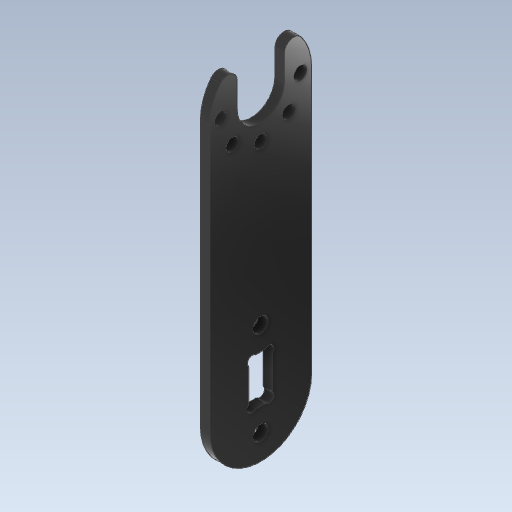
# Autodesk Inventor part: ForeArm_inside_frame
Saved by Autodesk Inventor 2020 (Build 240168000, 168)
## iProperties
Part Number: ForeArm_inside_frame
Material: GFRP
Document SubType Name: Modeling
Designer: Masato Kubotera
Density: 1.75 g/cm^3
Appearance: 低 光沢 - 黒
Description: GFRP T2
Mass: 4.75794 g
Surface Area: 33.053 cm^2
Volume: 2.71883 cm^3
Author: Masato Kubotera
Autodesk Inventor part; units mm, degrees
ref_plane "YZ Plane" through (0, 0, 0) normal (1, 0, 0) x (0, 1, 0)
ref_plane "XZ Plane" through (0, 0, 0) normal (0, 1, 0) x (-1, 0, 0)
ref_plane "XY Plane" through (0, 0, 0) normal (0, 0, 1) x (1, 0, 0)
derived "ForeArm_outside_frame.ipt"
sketch "スケッチ1" plane through (0, 0, 0) normal (0, 1, 0) x (-1, 0, 0)
  circle A0 centre (0, 0) radius 5.05
  line L0 (-8.5, 0) -> (8.5, 0) construction
  circle A1 centre (-8.5, 0) radius 1.35
  circle A2 centre (-6.0104, -6.0104) radius 1.35
  circle A3 centre (0, -8.5) radius 1.35
  circle A4 centre (6.0104, -6.0104) radius 1.35
  circle A5 centre (0, -145.8097) radius 16
  line L1 (0, 0) -> (0, -145.8097) construction
  arc A6 (-20.3699, -115.9088) -> (20.3699, -115.9088) centre (0, -145.8097) ccw
  circle A7 centre (-8.5, 0) radius 2.4 construction
  line L2 (-16, 31) -> (16, 31) construction
  line L3 (16, 31) -> (16, -12) construction
  line L4 (16, -12) -> (-16, -12) construction
  line L5 (-16, -12) -> (-16, 31) construction
  line L6 (-16, 31) -> (16, -12) construction
  line L7 (16, 31) -> (-16, -12) construction
  arc A8 (-16, 0) -> (-10.583, -12) centre (0, 0) ccw construction
  arc A9 (10.583, -12) -> (16, 0) centre (0, 0) ccw construction
  line L8 (-16, -107.6443) -> (-16, 0)
  line L9 (16, -107.6443) -> (16, 0)
  circle A10 centre (0, -82.5) radius 1.6
  line L10 (0, -145.8097) -> (-25.5832, -120.2265) construction
  circle A11 centre (-22.7548, -123.055) radius 4 construction
  circle A12 centre (-22.7548, -123.055) radius 1.6
  circle A13 centre (-22.7548, -168.5645) radius 1.6
  circle A14 centre (22.7548, -168.5645) radius 1.6
  circle A15 centre (22.7548, -123.055) radius 1.6
  line L11 (30.6064, -21.0119) -> (2.8936, -37.0119) construction
  line L12 (2.8936, -37.0119) -> (-18.6064, 0.2272) construction
  line L13 (-18.6064, 0.2272) -> (9.1064, 16.2272) construction
  line L14 (9.1064, 16.2272) -> (30.6064, -21.0119) construction
  line L15 (30.6064, -21.0119) -> (-18.6064, 0.2272) construction
  line L16 (2.8936, -37.0119) -> (9.1064, 16.2272) construction
  line L17 (16.75, -29.0119) -> (-4.75, 8.2272) construction
  circle A16 centre (0, -42.5) radius 1.6
  line L18 (-2.5, -47.5) -> (2.5, -47.5) construction
  line L19 (2.5, -47.5) -> (2.5, -57.5) construction
  line L20 (2.5, -57.5) -> (-2.5, -57.5) construction
  line L21 (-2.5, -57.5) -> (-2.5, -47.5) construction
  line L22 (-2.5, -47.5) -> (2.5, -57.5) construction
  line L23 (2.5, -47.5) -> (-2.5, -57.5) construction
  line L24 (-2.5, -52.5) -> (2.5, -52.5) construction
  circle A17 centre (0, -62.5) radius 1.6
  line L25 (2.8936, -37.0119) -> (49.2811, -117.3573) construction
  line L26 (0, -145.8097) -> (49.2811, -117.3573) construction
  line L27 (-2.5, -47.5) -> (2.5, -47.5) construction
  line L28 (2.5, -47.5) -> (2.5, -77.5) construction
  line L29 (2.5, -77.5) -> (-2.5, -77.5) construction
  line L30 (-2.5, -77.5) -> (-2.5, -47.5) construction
  line L31 (-2.5, -47.5) -> (2.5, -77.5) construction
  line L32 (2.5, -47.5) -> (-2.5, -77.5) construction
  line L33 (-2.55, -47.45) -> (2.55, -47.45)
  line L34 (2.55, -47.45) -> (2.55, -77.55)
  line L35 (2.55, -77.55) -> (-2.55, -77.55)
  line L36 (-2.55, -77.55) -> (-2.55, -47.45)
  line L37 (-2.55, -47.45) -> (2.55, -77.55) construction
  line L38 (2.55, -47.45) -> (-2.55, -77.55) construction
  arc A18 (-1.0651, -47.45) -> (-2.55, -48.9349) centre (-1.8075, -48.1925) ccw
  arc A19 (2.55, -48.9349) -> (1.0651, -47.45) centre (1.8075, -48.1925) ccw
  line L39 (-2.5, -62.5) -> (2.5, -62.5) construction
  arc A20 (-2.55, -76.0651) -> (-1.0651, -77.55) centre (-1.8075, -76.8075) ccw
  arc A21 (1.0651, -77.55) -> (2.55, -76.0651) centre (1.8075, -76.8075) ccw
  arc A22 (16, 0) -> (8.0571, 13.8233) centre (0, 0) ccw
  circle A23 centre (0, -145.8097) radius 28.1801
  line L40 (-5.05, 0) -> (-5.05, 12.0954)
  line L41 (5.05, 0) -> (5.05, 12.0954)
  circle A24 centre (8.5, 0) radius 1.35
  arc A25 (-8.0571, 13.8233) -> (-16, 0) centre (0, 0) ccw
  arc A26 (-5.05, 12.0954) -> (-8.0571, 13.8233) centre (-7.05, 12.0954) ccw
  arc A27 (8.0571, 13.8233) -> (5.05, 12.0954) centre (7.05, 12.0954) ccw
  arc A28 (-20.3699, -115.9088) -> (-16, -107.6443) centre (-26, -107.6443) ccw
  arc A29 (16, -107.6443) -> (20.3699, -115.9088) centre (26, -107.6443) ccw
  point P0 (0, 9.5)
  point P1 (0, 9.5)
  point P2 (-16, -113.3598)
  point P3 (16, -113.3598)
  point P4 (6, -10.3923)
  point P5 (0, -52.5)
  point P6 (0, -62.5)
  point P7 (0, -181.9899)
  point P8 (-5.05, 15.1821)
  point P9 (5.05, 15.1821)
  point P10 (1.0651, -77.55)
  point P11 (-1.0651, -77.55)
  point P12 (-2.55, -76.0651)
  point P13 (2.55, -48.9349)
  point P14 (2.55, -76.0651)
  point P15 (5.05, 9.6596)
  point P16 (5.05, 0)
sketch "スケッチ2" plane through (0, 0, 0) normal (0, 1, 0) x (-1, 0, 0)
  line L0 (-2.55, -77.55) -> (-2.55, -47.45) projected
  line L1 (2.55, -47.45) -> (2.55, -77.55) projected
  line L2 (2.5, -57.5) -> (-2.5, -57.5) construction
  arc A0 (-1.0651, -47.45) -> (-2.55, -48.9349) centre (-1.8075, -48.1925) ccw projected
  arc A1 (2.55, -48.9349) -> (1.0651, -47.45) centre (1.8075, -48.1925) ccw projected
  line L3 (-2.55, -47.45) -> (2.55, -47.45) projected
  line L4 (-2.55, -57.55) -> (2.55, -57.55)
  line L5 (-2.5, -57.5) -> (-2.5, -47.5) construction
  arc A2 (-2.55, -56.0651) -> (-1.0651, -57.55) centre (-1.8075, -56.8075) ccw
  line L6 (0, 0) -> (0, -145.8097) construction
  arc A3 (1.0651, -57.55) -> (2.55, -56.0651) centre (1.8075, -56.8075) ccw
  circle A4 centre (0, -62.5) radius 1.6 projected
  arc A5 (-10.9, -56.8906) -> (10.9, -56.8906) centre (0, -56.8906) ccw
  line L7 (-16, -113.3598) -> (-16, 0) projected
  line L8 (16, -113.3598) -> (16, 0) projected
  arc A6 (16, 0) -> (-16, 0) centre (0, 0) ccw projected
  circle A7 centre (-8.5, 0) radius 1.35 projected
  circle A8 centre (-6.0104, -6.0104) radius 1.35 projected
  circle A9 centre (0, 0) radius 5.05 projected
  circle A10 centre (0, -8.5) radius 1.35 projected
  circle A11 centre (6.0104, -6.0104) radius 1.35 projected
  circle A12 centre (0, -42.5) radius 1.6 projected
  line L9 (-2.5, -37.5) -> (2.5, -37.5) construction
  line L10 (2.5, -37.5) -> (2.5, -67.5) construction
  line L11 (2.5, -67.5) -> (-2.5, -67.5) construction
  line L12 (-2.5, -67.5) -> (-2.5, -37.5) construction
  line L13 (-2.5, -37.5) -> (2.5, -67.5) construction
  line L14 (2.5, -37.5) -> (-2.5, -67.5) construction
  line L15 (-2.5, -52.5) -> (2.5, -52.5) construction
  arc A13 (-5.05, 12.0954) -> (-8.0571, 13.8233) centre (-7.05, 12.0954) ccw projected
  line L16 (-5.05, 0) -> (-5.05, 12.0954) projected
  arc A14 (8.0571, 13.8233) -> (5.05, 12.0954) centre (7.05, 12.0954) ccw projected
  line L17 (5.05, 0) -> (5.05, 12.0954) projected
  circle A15 centre (8.5, 0) radius 1.35 projected
  line L18 (-10.9, -56.8906) -> (-10.9, 0)
  line L19 (10.9, -56.8906) -> (10.9, 0)
  arc A16 (-8.6343, 6.6528) -> (-10.9, 0) centre (0, 0) ccw
  arc A17 (10.9, 0) -> (8.6343, 6.6528) centre (0, 0) ccw
  line L20 (-5.05, 5.4321) -> (-5.05, 0)
  line L21 (5.05, 5.4321) -> (5.05, 0)
  arc A18 (-5.05, 5.4321) -> (-8.6343, 6.6528) centre (-7.05, 5.4321) ccw
  arc A19 (8.6343, 6.6528) -> (5.05, 5.4321) centre (7.05, 5.4321) ccw
  circle A20 centre (-8.5, 0) radius 2.4 construction
  point P0 (1.0651, -57.55)
  point P1 (2.55, -56.0651)
  point P2 (0, -52.5)
  point P3 (0, -52.5)
  point P4 (-2.55, -67.4881)
  point P5 (2.55, -67.4881)
  point P6 (-5.05, 9.6596)
  point P7 (5.05, 9.6596)
  dimension "d6" = 0.05
  dimension "d7" = 0.05
  dimension "d8" = 1.05
  dimension "d9" = 1.05
  dimension "d13" = 5
  dimension "d14" = 30
  dimension "d15" = 2
  dimension "d17" = 4.8
  constraints: 22 end point, 18 point on circle, 10 tangent, 9 point on line, 8 centre point, 5 symmetric about line, 4 midpoint, 4 parallel, 2 coincident, 2 perpendicular, 1 collinear, 1 equal radius, 1 horizontal, 1 vertical, 3 other
  measures "d6" distance between parallel lines of L4 L2
  measures "d7" distance between parallel lines of L0 L5
  measures "d8" radius of A2
  measures "d9" radius of A0
  measures "d13" distance of L10.end L11.end
  measures "d14" distance of L9.end L10.end
  measures "d15" radius of A18
  measures "d17" diameter of A20
extrude "押し出し1" add sketch "スケッチ2" along normal blind 2 contours A2 L4 A3 L1 A5 L0 | L0 A5 L18 A16 A18 L16 A9 L17 A19 A17 L19 L1 A3 A1 L3 A0 A2
equation "\"d6\" = d7"
equation "\"d8\" = d9"
